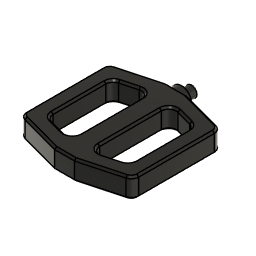
pedal (Autodesk Fusion 360 design; units mm, degrees)
Autodesk Fusion 360 part; units mm, degrees
note: some values were not read from the file. Chosen so that the rebuilt part matches the saved one: which face or edge a step refers to.
sketch "base" plane through (0, 0, 0) normal (0, 0, 1) x (1, 0, 0) in component "pedal"
  line L0 (45, 45) -> (-45, 45)
  line L1 (-45, 45) -> (-45, -45)
  line L2 (-45, -45) -> (45, -45)
  line L3 (45, -45) -> (45, 45)
  line L4 (45, 45) -> (-45, -45) construction
  line L5 (-45, 45) -> (45, -45) construction
  line L6 (-45, 45) -> (45, 45) construction
  line L7 (45, 45) -> (45, 35) construction
  line L8 (45, 35) -> (-45, 35) construction
  line L9 (-45, 35) -> (-45, 45) construction
  line L10 (-45, 35) -> (45, 35) construction
  line L11 (45, 35) -> (45, -35)
  line L12 (45, -35) -> (-45, -35) construction
  line L13 (-45, -35) -> (-45, 35)
  line L14 (8, 45) -> (-8, 45)
  line L15 (-8, 45) -> (-8, -45)
  line L16 (-8, -45) -> (8, -45)
  line L17 (8, -45) -> (8, 45)
  line L18 (8, 45) -> (-8, -45) construction
  line L19 (-8, 45) -> (8, -45) construction
  line L20 (-45, 35) -> (-8, 45)
  line L21 (8, 45) -> (45, 35)
  line L22 (45, -35) -> (8, -45)
  line L23 (-8, -45) -> (-45, -35)
  line L24 (-4.8691, -33.4156) -> (-33, -25.8127)
  line L25 (-33, -25.8127) -> (-33, 25.8127)
  line L26 (-33, 25.8127) -> (-4.8691, 33.4156)
  line L27 (4.8691, 33.4156) -> (33, 25.8127)
  line L28 (33, 25.8127) -> (33, -25.8127)
  line L29 (33, -25.8127) -> (4.8691, -33.4156)
  dimension "d1" = 90
  dimension "d2" = 90
  dimension "d3" = 90
  dimension "d4" = 10
  dimension "d5" = 90
  dimension "d6" = 70
  dimension "d7" = 16
  dimension "d8" = 90
  dimension "d9" = 12
  dimension "d10" = 12
  constraint horizontal L0
  constraint perpendicular L0 L1
  constraint parallel L0 L2
  constraint parallel L1 L3
  constraint coincident L4 origin
  constraint coincident L5 origin
  constraint horizontal L6
  constraint vertical L7
  constraint horizontal L8
  constraint vertical L9
  constraint horizontal L10
  constraint vertical L11
  constraint horizontal L12
  constraint vertical L13
  constraint horizontal L14
  constraint perpendicular L14 L15
  constraint parallel L14 L16
  constraint parallel L15 L17
  constraint coincident L18 origin
  constraint coincident L19 origin
  measures "d1" distance of L1.end L2.end
  measures "d2" distance of L0.end L1.end
  measures "d3" distance of L0.end L0.start
  measures "d4" distance of L0.end L8.end
  measures "d5" distance of L8.end L7.end
  measures "d6" distance of L8.end L12.end
  measures "d7" distance of L15.end L16.end
  measures "d8" distance of L14.end L15.end
extrude "Extrude1" add sketch "base" along normal blind 16 contours L0 L2 L14 L15 L16 L17 | L3 L11 L17 L21 L22 L27 L28 L29 | L1 L13 L15 L20 L23 L24 L25 L26 in component "pedal"
fillet "Fillet1" radius 6 4 edges at (-45, -35, 8) (-45, 35, 8) (45, 35, 8) (45, -35, 8) in component "pedal"
fillet "Fillet3" radius 6 8 edges at (-33, 25.8127, 8) (-33, -25.8127, 8) (-8, 32.5694, 8) (-8, -32.5694, 8) (8, -32.5694, 8) (8, 32.5694, 8) (33, 25.8127, 8) (33, -25.8127, 8) in component "pedal"
sketch "extension" plane through (0, 45, 0) normal (0, 1, 0) x (-1, 0, 0) in component "pedal"
  line L0 (8, 0) -> (8, 16)
  line L1 (-8, 16) -> (-8, 0)
  line L2 (-8, 0) -> (8, 16) construction
  line L3 (-8, 16) -> (8, 0) construction
  circle A0 centre (0, 8) radius 8
  circle A1 centre (0, 8) radius 4.425
  line L4 (-8, 0) -> (8, 0)
  line L5 (8, 16) -> (-8, 16)
  dimension "d19" = 16
  dimension "d25" = 8.85
  constraint coincident L1.end L2.start
  constraint coincident L0.end L2.end
  constraint coincident L1.start L3.start
  constraint coincident L0.start L3.end
  constraint midpoint L3 A0.centre
  constraint concentric A0 A1
  measures "d19" diameter of A0
  measures "d25" diameter of A1
extrude "Extrude3" add sketch "extension" along normal blind 12 contours A1 in component "pedal"
extrude "Extrude4" add sketch "extension" along normal blind 4 contours A0 in component "pedal"
chamfer "Chamfer1" distance 1.5 angle 45 58 edges at (-4, 45, 0) (4, 45, 0) (-4, 45, 16) (8, 0, 0) (10.3526, -29.4966, 0) (10.3526, 29.4966, 0) (22.0655, -28.768, 0) (22.0655, 28.768, 0) (31.7641, -24.8665, 0) (31.7641, 24.8665, 0) (33, 0, 0) (24.2827, -40.5993, 0) (43.7641, -34.0538, 0) (0, -45, 0) (45, 0, 0) (-24.2827, -40.5993, 0) (43.7641, 34.0538, 0) (-43.7641, -34.0538, 0) (24.2827, 40.5993, 0) (-45, 0, 0) (-43.7641, 34.0538, 0) (-24.2827, 40.5993, 0) (-8, 0, 0) (-10.3526, 29.4966, 0) (-10.3526, -29.4966, 0) (-22.0655, 28.768, 0) (-22.0655, -28.768, 0) (-31.7641, 24.8665, 0) (-31.7641, -24.8665, 0) (-33, 0, 0) (-24.2827, 40.5993, 16) (4, 45, 16) (24.2827, 40.5993, 16) (8, 0, 16) (10.3526, -29.4966, 16) (10.3526, 29.4966, 16) (22.0655, -28.768, 16) (22.0655, 28.768, 16) (31.7641, -24.8665, 16) (31.7641, 24.8665, 16) (33, 0, 16) (24.2827, -40.5993, 16) (43.7641, -34.0538, 16) (0, -45, 16) (45, 0, 16) (-24.2827, -40.5993, 16) (43.7641, 34.0538, 16) (-43.7641, -34.0538, 16) (-45, 0, 16) (-43.7641, 34.0538, 16) (-8, 0, 16) (-10.3526, 29.4966, 16) (-10.3526, -29.4966, 16) (-22.0655, 28.768, 16) (-22.0655, -28.768, 16) (-31.7641, 24.8665, 16) (-31.7641, -24.8665, 16) (-33, 0, 16) in component "pedal"
component "pedal" placed x (1, 0, 0) y (0, 1, 0) z (0, 0, 1) at (0, 0, 0)
equation "d28 = 12 mm - 8 mm"
named bodies: "pedal"
